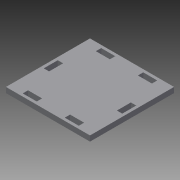
# Autodesk Inventor part: bottom
Saved by Autodesk Inventor 2015 SP1 (Build 190203100, 203)
## iProperties
Created: 2016-04-13
Part Number: bottom
Material: Generic
Document SubType Name: Modeling
Designer: tuttlem
Density: 1 g/cm^3
Appearance: Default
Author: tuttlem
Autodesk Inventor part; units mm, degrees
ref_plane "YZ Plane" through (0, 0, 0) normal (1, 0, 0) x (0, 1, 0)
ref_plane "XZ Plane" through (0, 0, 0) normal (0, 1, 0) x (-1, 0, 0)
ref_plane "XY Plane" through (0, 0, 0) normal (0, 0, 1) x (1, 0, 0)
sketch "Sketch1" plane through (0, 0, 0) normal (0, 1, 0) x (-1, 0, 0)
  line L0 (0, 0) -> (-76.2, 0)
  line L1 (-76.2, 0) -> (-76.2, -76.2)
  line L2 (-76.2, -76.2) -> (0, -76.2)
  line L3 (0, -76.2) -> (0, 0)
  line L4 (-12.7, -2.54) -> (-25.4, -2.54)
  line L5 (-25.4, -2.54) -> (-25.4, -7.366)
  line L6 (-25.4, -7.366) -> (-12.7, -7.366)
  line L7 (-12.7, -7.366) -> (-12.7, -2.54)
  line L8 (-38.1, 0) -> (-38.1, -76.2)
  line L9 (0, -38.1) -> (-76.2, -38.1)
  line L10 (-12.7, -73.66) -> (-25.4, -73.66)
  line L11 (-25.4, -73.66) -> (-25.4, -68.834)
  line L12 (-25.4, -68.834) -> (-12.7, -68.834)
  line L13 (-12.7, -68.834) -> (-12.7, -73.66)
  line L14 (-63.5, -2.54) -> (-50.8, -2.54)
  line L15 (-50.8, -2.54) -> (-50.8, -7.366)
  line L16 (-50.8, -7.366) -> (-63.5, -7.366)
  line L17 (-63.5, -7.366) -> (-63.5, -2.54)
  line L18 (-63.5, -73.66) -> (-50.8, -73.66)
  line L19 (-50.8, -73.66) -> (-50.8, -68.834)
  line L20 (-50.8, -68.834) -> (-63.5, -68.834)
  line L21 (-63.5, -68.834) -> (-63.5, -73.66)
  line L22 (-68.834, -31.75) -> (-68.834, -44.45)
  line L23 (-68.834, -44.45) -> (-73.66, -44.45)
  line L24 (-73.66, -31.75) -> (-68.834, -31.75)
  line L25 (-73.66, -44.45) -> (-73.66, -31.75)
  line L26 (-7.366, -44.45) -> (-2.54, -44.45)
  line L27 (-7.366, -31.75) -> (-7.366, -44.45)
  line L28 (-2.54, -44.45) -> (-2.54, -31.75)
  line L29 (-2.54, -31.75) -> (-7.366, -31.75)
  dimension "d0" = 76.2
  dimension "d1" = 76.2
  dimension "d2" = 12.7
  dimension "d3" = 4.826
  dimension "d4" = 2.54
  dimension "d5" = 12.7
  dimension "d6" = 31.75
  dimension "d7" = 2.54
  dimension "d8" = 4.826
  dimension "d9" = 12.7
  constraints: 60 end point, 16 symmetric about line, 4 midpoint, 4 parallel, 2 horizontal, 2 perpendicular
  measures "d0" distance of L2.end L1.end
  measures "d1" distance of L1.end L0.end
  measures "d2" distance of L6.end L5.end
  measures "d3" distance of L5.end L4.end
  measures "d4" distance between parallel lines of L0 L4
  measures "d5" distance between parallel lines of L3 L7
  measures "d6" distance from line of L24 L0.end
  measures "d7" distance between parallel lines of L25 L1
  measures "d8" distance of L23.start L23.end
  measures "d9" distance of L22.start L23.start
extrude "Extrusion1" add sketch "Sketch1" along normal blind 4.826 contours L3 L9 L28 L29 L27 L8 L0 | L8 L9 L22 L24 L25 L1 L0 | L3 L2 L8 L9 L27 L26 L28 | L8 L2 L1 L9 L25 L23 L22
body "Solid1"
